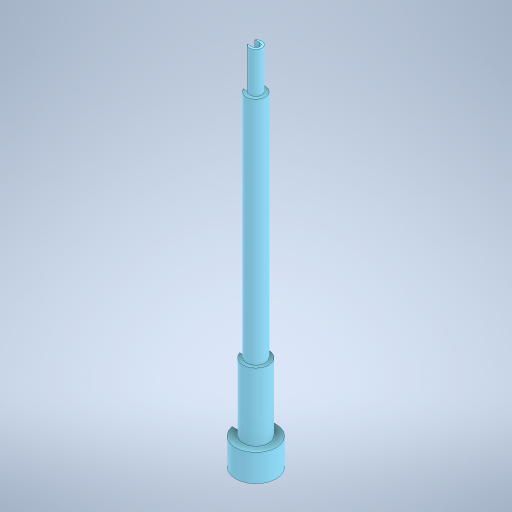
# Autodesk Inventor part: Norhof wire channel top
Saved by Autodesk Inventor 2023 (Build 270158030, 158C)
## iProperties
Created: 2022-09-08
Part Number: Norhof wire channel top
Material: Generic
Document SubType Name: Modeling
Designer: Julian
Density: 1 g/cm^3
Appearance: Default
Author: Julian
Autodesk Inventor part; units mm, degrees
ref_plane "YZ Plane" through (0, 0, 0) normal (1, 0, 0) x (0, 1, 0)
ref_plane "XZ Plane" through (0, 0, 0) normal (0, 1, 0) x (-1, 0, 0)
ref_plane "XY Plane" through (0, 0, 0) normal (0, 0, 1) x (1, 0, 0)
sketch "Sketch1" plane through (0, 0, 0) normal (0, 1, 0) x (-1, 0, 0)
  circle A0 centre (0, 0) radius 3.5
  circle A1 centre (0, 0) radius 2.25
  circle A2 centre (0, 0) radius 1.4
  line L0 (0, 0) -> (-1.4, 0)
  line L1 (-1.4, 0) -> (-1.4, -1.4)
  line L2 (-1.4, -1.4) -> (0, -1.4)
  line L3 (0, -1.4) -> (0, 0)
  line L4 (-1.4, -1.4) -> (7.6159, -1.4)
  line L5 (7.6159, -1.4) -> (7.6159, 1.4)
  line L6 (7.6159, 1.4) -> (-1.4, 1.4)
  line L7 (-1.4, 1.4) -> (-1.4, -1.4)
  point P0 (0, 1.4)
  point P1 (3.2078, 1.4)
  point P2 (3.2078, -1.4)
  point P3 (1.7614, 1.4)
  point P4 (1.7614, -1.4)
  dimension "d0" = 7
  dimension "d1" = 4.5
  dimension "d6" = 2.8
  constraints: 16 end point, 4 parallel, 3 centre point, 3 coincident, 2 horizontal, 2 perpendicular
  measures "d0" diameter of A0
  measures "d1" diameter of A1
  measures "d6" diameter of A2
extrude "Extrusion1" add sketch "Sketch1" against normal blind 110 contours L6 A1 L4 A0 | L6 L7 L1 L2 L4 A1 | A2 L7 L6 | L2 L1 A2 picked at (2.5783, 1.6484)
extrude "Extrusion2" add sketch "Sketch1" along normal blind 15 contours L6 L7 L1 L2 L4 A1 | A2 L7 L6 | L2 L1 A2
sketch "Sketch2" plane through (0, -110, 0) normal (0, -1, 0) x (1, 0, 0)
  circle A0 centre (0, 0) radius 4.75
  circle A1 centre (0, 0) radius 7.5
  arc A2 (-3.2078, -1.4) -> (-3.2078, 1.4) centre (0, 0) ccw projected
  line L0 (-3.2078, 1.4) -> (0, 1.4) projected
  arc A3 (0, -1.4) -> (0, 1.4) centre (0, 0) ccw projected
  line L1 (0, -1.4) -> (-3.2078, -1.4) projected
  line L2 (1.4, -1.4) -> (-7.6159, -1.4) projected
  line L3 (-7.6159, 1.4) -> (1.4, 1.4) projected
  point P0 (-4.539, 1.4)
  point P1 (-4.539, -1.4)
  point P2 (-7.3682, 1.4)
  point P3 (-7.3682, -1.4)
  dimension "d7" = 9.5
  dimension "d8" = 15
  constraints: 2 centre point, 2 coincident
  measures "d7" diameter of A0
  measures "d8" diameter of A1
extrude "Extrusion3" add sketch "Sketch2" against normal blind 25 contours A0 L2 A2 L3
extrude "Extrusion4" add sketch "Sketch2" along normal blind 10 contours A0 L2 A2 L3 | A0 L3 A1 L2 | A2 L1 A3 L0 picked at (6.4638, 0.9807)
body "Solid1"
